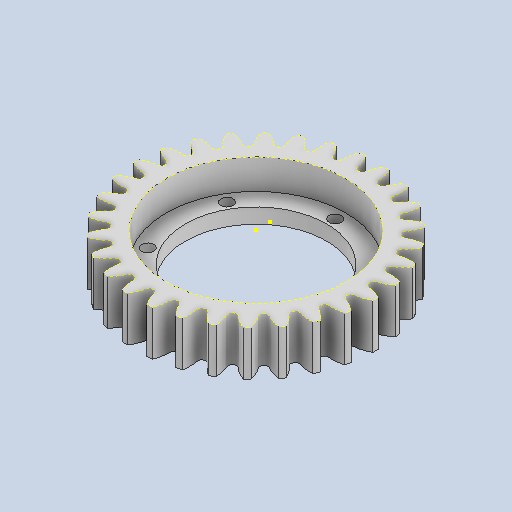
# Autodesk Inventor part: ZubkataiaBig
Saved by Autodesk Inventor 2024 (Build 280153000, 153)
## iProperties
Created: 2023-10-17
Part Number: ZubkataiaBig
Material: Generic
Document SubType Name: Modeling
Designer: Kippi
Density: 1 g/cm^3
Appearance: Default
Author: Kippi
Autodesk Inventor part; units mm, degrees
ref_plane "YZ Plane" through (0, 0, 0) normal (1, 0, 0) x (0, 1, 0)
ref_plane "XZ Plane" through (0, 0, 0) normal (0, 1, 0) x (-1, 0, 0)
ref_plane "XY Plane" through (0, 0, 0) normal (0, 0, 1) x (1, 0, 0)
sketch "Sketch1" plane through (0, 0, 0) normal (0, 1, 0) x (-1, 0, 0)
  circle A0 centre (0.0407, 9.5963) radius 62.5
  circle A1 centre (0.0407, 9.5963) radius 53
  circle A2 centre (0.0407, -43.4037) radius 4.05
  circle A3 centre (0.0407, 9.5963) radius 44
  circle A4 centre (45.9401, -16.9037) radius 4.05
  circle A5 centre (45.9401, 36.0963) radius 4.05
  circle A6 centre (0.0407, 62.5963) radius 4.05
  circle A7 centre (-45.8586, 36.0963) radius 4.05
  circle A8 centre (-45.8586, -16.9037) radius 4.05
  circle A9 centre (0.0407, 9.5963) radius 47.2699
  circle A10 centre (0.0407, 9.5963) radius 79.9939
  point P0 (0, 0)
  dimension "d3" = 106
  dimension "d2" = 125
  dimension "d4" = 360
  dimension "d5" = 8.1
  constraints: 10 centre point, 5 coincident, 1 vertical alignment, 15 other
  measures "d2" diameter of A0
  measures "d5" diameter of A2
extrude "Extrusion1" add sketch "Sketch1" along normal blind 30 contours A0 | A1 A4 A2 A8 A7 A6 A5 | A10
sketch "Sketch2" plane through (-0.0407, 30, 9.5963) normal (0, 1, 0) x (1, 0, 0)
  circle A0 centre (0, 0) radius 47.2699 construction
  circle A1 centre (0, 0) radius 60
  point P0 (0.0407, 9.5963)
  dimension "d8" = 120
  constraints: 1 centre point, 1 coincident
  measures "d8" diameter of A1
extrude "Extrusion2" cut sketch "Sketch2" against normal blind 20
sketch "Sketch4" plane through (-0.0407, 30, 9.5963) normal (0, 1, 0) x (1, 0, 0)
  spline S0 degree 3 poles (-6.5259, 79.7334) (-6.2263, 79.2581) (-5.7769, 78.5452) (-5.2243, 77.5668) (-4.8273, 76.8235) (-4.451, 76.0694) (-4.0967, 75.3048) (-3.7666, 74.5294) (-3.4631, 73.7432) (-3.1905, 72.9457) (-2.9506, 72.1376) (-2.7945, 71.4528) (-2.6817, 70.9025) (-2.5626, 70.4977) (-2.4016, 70.1077) (-2.1917, 69.7409) (-1.9706, 69.4668) (-1.7708, 69.2687) (-1.6019, 69.1425) (-1.4288, 69.0215) (-1.2381, 68.9312) (-1.0444, 68.8474) (-0.8391, 68.7979) (-0.6323, 68.7561) (-0.3509, 68.7461) (0, 68.7526) (0.3509, 68.7461) (0.6323, 68.7561) (0.8391, 68.7979) (1.0444, 68.8474) (1.2381, 68.9312) (1.4288, 69.0215) (1.6019, 69.1425) (1.7708, 69.2687) (1.9706, 69.4668) (2.1917, 69.7409) (2.4016, 70.1077) (2.5626, 70.4977) (2.6817, 70.9025) (2.7945, 71.4528) (2.9506, 72.1376) (3.1905, 72.9457) (3.4631, 73.7432) (3.7666, 74.5294) (4.0967, 75.3048) (4.451, 76.0694) (4.8273, 76.8235) (5.2243, 77.5668) (5.7769, 78.5452) (6.2263, 79.2581) (6.5259, 79.7334) knots 0 0 0 0 0.168512 0.252773 0.337035 0.421295 0.505556 0.589816 0.674075 0.758333 0.842588 0.926838 0.968959 1.011074 1.053192 1.095291 1.137378 1.158442 1.179505 1.200561 1.221628 1.242684 1.263747 1.284807 1.305869 1.348 1.390132 1.411193 1.432253 1.453316 1.474372 1.495439 1.516495 1.537558 1.558622 1.60071 1.642808 1.684926 1.727041 1.769162 1.853412 1.937667 2.021925 2.106184 2.190444 2.274705 2.358966 2.443227 2.527488 2.696 2.696 2.696 2.696
  circle A0 centre (0, 0) radius 68.75 construction
  circle A1 centre (0, 0) radius 70.4769 construction
  circle A2 centre (0, 0) radius 75 construction
  circle A3 centre (0, 0) radius 80
  point P0 (0.0407, 9.5963)
  point P1 (-5.6426, 78.2983)
  point P2 (-5.2272, 77.5652)
  point P3 (-4.8307, 76.8217)
  point P4 (-4.4547, 76.0677)
  point P5 (-4.1007, 75.303)
  point P6 (-3.771, 74.5276)
  point P7 (-3.4682, 73.7413)
  point P8 (-3.1959, 72.9439)
  point P9 (-2.9594, 72.1353)
  point P10 (-2.7673, 71.315)
  point P11 (-2.676, 70.9038)
  point P12 (-2.5556, 70.5002)
  point P13 (-2.3934, 70.1115)
  point P14 (-2.1825, 69.7472)
  point P15 (-1.9188, 69.4191)
  point P16 (-1.7676, 69.2724)
  point P17 (-1.6012, 69.1434)
  point P18 (-1.4259, 69.0267)
  point P19 (-1.2376, 68.9322)
  point P20 (-1.0425, 68.8531)
  point P21 (-0.8389, 68.7992)
  point P22 (-0.6316, 68.7618)
  point P23 (-0.4213, 68.7499)
  point P24 (0, 68.75)
  point P25 (0.4213, 68.7499)
  point P26 (0.6316, 68.7618)
  point P27 (0.8389, 68.7992)
  point P28 (1.0425, 68.8531)
  point P29 (1.2376, 68.9322)
  point P30 (1.4259, 69.0267)
  point P31 (1.6012, 69.1434)
  point P32 (1.7676, 69.2724)
  point P33 (1.9188, 69.4191)
  point P34 (2.1825, 69.7472)
  point P35 (2.3934, 70.1115)
  point P36 (2.5556, 70.5002)
  point P37 (2.676, 70.9038)
  point P38 (2.7673, 71.315)
  point P39 (2.9594, 72.1353)
  point P40 (3.1959, 72.9439)
  point P41 (3.4682, 73.7413)
  point P42 (3.771, 74.5276)
  point P43 (4.1007, 75.303)
  point P44 (4.4547, 76.0677)
  point P45 (4.8307, 76.8217)
  point P46 (5.2272, 77.5652)
  point P47 (5.6426, 78.2983)
  constraints: 4 centre point, 2 point on circle, 49 other
extrude "Extrusion3" cut sketch "Sketch4" against normal blind 30 contours A3 S0 picked at (-0.4798, 76.1142)
pattern_circular "Circular Pattern1" count 30 over 360 about axis through (-0.0407, 30, 9.5963) along (0, -1, 0) of "Extrusion3"
sketch "Sketch5" plane through (0, 30, 0) normal (0, 1, 0) x (1, 0, 0)
  circle A0 centre (-0.0407, -9.5963) radius 60 construction
  arc A1 (-22.9968, 67.033) -> (-26.5105, 65.8913) centre (-0.0407, -9.5963) ccw construction
  arc A2 (-38.4272, 60.5856) -> (-41.6268, 58.7384) centre (-0.0407, -9.5963) ccw construction
  arc A3 (-52.18, 51.071) -> (-54.9256, 48.5989) centre (-0.0407, -9.5963) ccw construction
  arc A4 (-63.6541, 38.9049) -> (-65.8257, 35.9159) centre (-0.0407, -9.5963) ccw construction
  arc A5 (-72.3479, 24.6191) -> (-73.8507, 21.2439) centre (-0.0407, -9.5963) ccw construction
  arc A6 (-77.8816, 8.8379) -> (-78.6498, 5.2241) centre (-0.0407, -9.5963) ccw construction
  arc A7 (-80.0133, -7.749) -> (-80.0133, -11.4435) centre (-0.0407, -9.5963) ccw construction
  arc A8 (-78.6498, -24.4166) -> (-77.8816, -28.0304) centre (-0.0407, -9.5963) ccw construction
  arc A9 (-73.8507, -40.4365) -> (-72.3479, -43.8116) centre (-0.0407, -9.5963) ccw construction
  arc A10 (-65.8257, -55.1085) -> (-63.6541, -58.0974) centre (-0.0407, -9.5963) ccw construction
  arc A11 (-54.9256, -67.7914) -> (-52.18, -70.2635) centre (-0.0407, -9.5963) ccw construction
  arc A12 (-41.6268, -77.9309) -> (-38.4272, -79.7782) centre (-0.0407, -9.5963) ccw construction
  arc A13 (-26.5105, -85.0838) -> (-22.9968, -86.2255) centre (-0.0407, -9.5963) ccw construction
  arc A14 (-10.2373, -88.9376) -> (-6.563, -89.3238) centre (-0.0407, -9.5963) ccw construction
  arc A15 (6.4815, -89.3238) -> (10.1558, -88.9376) centre (-0.0407, -9.5963) ccw construction
  arc A16 (22.9153, -86.2255) -> (26.429, -85.0838) centre (-0.0407, -9.5963) ccw construction
  arc A17 (38.3457, -79.7782) -> (41.5453, -77.9309) centre (-0.0407, -9.5963) ccw construction
  arc A18 (52.0985, -70.2635) -> (54.8441, -67.7914) centre (-0.0407, -9.5963) ccw construction
  arc A19 (63.5726, -58.0974) -> (65.7442, -55.1085) centre (-0.0407, -9.5963) ccw construction
  arc A20 (72.2665, -43.8116) -> (73.7692, -40.4365) centre (-0.0407, -9.5963) ccw construction
  arc A21 (77.8001, -28.0304) -> (78.5683, -24.4166) centre (-0.0407, -9.5963) ccw construction
  arc A22 (79.9318, -11.4435) -> (79.9318, -7.749) centre (-0.0407, -9.5963) ccw construction
  arc A23 (78.5683, 5.2241) -> (77.8001, 8.8379) centre (-0.0407, -9.5963) ccw construction
  arc A24 (73.7692, 21.2439) -> (72.2665, 24.6191) centre (-0.0407, -9.5963) ccw construction
  arc A25 (65.7442, 35.9159) -> (63.5726, 38.9049) centre (-0.0407, -9.5963) ccw construction
  arc A26 (54.8441, 48.5989) -> (52.0985, 51.071) centre (-0.0407, -9.5963) ccw construction
  arc A27 (41.5453, 58.7384) -> (38.3457, 60.5856) centre (-0.0407, -9.5963) ccw construction
  arc A28 (26.429, 65.8913) -> (22.9153, 67.033) centre (-0.0407, -9.5963) ccw construction
  arc A29 (10.1558, 69.7451) -> (6.4815, 70.1313) centre (-0.0407, -9.5963) ccw construction
  arc A30 (-6.563, 70.1313) -> (-10.2373, 69.7451) centre (-0.0407, -9.5963) ccw construction
  point P0 (0, 0)
  constraints: 2 horizontal alignment, 28 other
body "Solid1"
